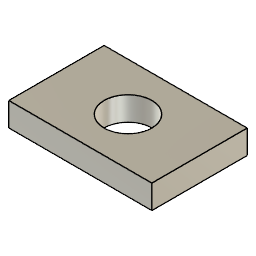
fixture-inch-job (Autodesk Fusion 360 design; units mm, degrees)
part number: 2026-04-07-15-25-03-247
Autodesk Fusion 360 part; units mm, degrees
sketch "RectangleWithCircle" plane through (0, 0, 0) normal (0, 0, 1) x (1, 0, 0)
  line L0 (-38.1, -25.4) -> (38.1, -25.4)
  line L1 (38.1, -25.4) -> (38.1, 25.4)
  line L2 (38.1, 25.4) -> (-38.1, 25.4)
  line L3 (-38.1, 25.4) -> (-38.1, -25.4)
  circle A0 centre (0, 0) radius 12.7
  dimension "d1" = 76.2
  dimension "d2" = 50.8
  dimension "d3" = 25.4
  measures "d1" horizontal distance of L0.start L0.end
  measures "d2" vertical distance of L0.end L1.end
  measures "d3" diameter of A0
sketch "Sketch2" plane through (0, 0, 0) normal (0, 0, 1) x (1, 0, 0)
  line L0 (-38.1, -25.4) -> (38.1, -25.4)
  line L1 (38.1, -25.4) -> (38.1, 25.4)
  line L2 (38.1, 25.4) -> (-38.1, 25.4)
  line L3 (-38.1, 25.4) -> (-38.1, -25.4)
  dimension "d6" = 50.8
  dimension "d7" = 76.2
  constraint coincident L0.end L1.start
  constraint coincident L1.end L2.start
  constraint coincident L2.end L3.start
  constraint coincident L0.start L3.end
  constraint parallel L0 L2
  constraint parallel L1 L3
  constraint perpendicular L0 L1
  measures "d6" distance of L0 L2
  measures "d7" distance of L1 L3
extrude "Extrude1" add sketch "Sketch2" along normal blind 12.7
extrude "Extrude2" cut sketch "RectangleWithCircle" along normal through all contours A0
equation "d3 = ( 1.27 cm ) * 2"
